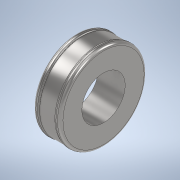
# Autodesk Inventor part: f8-16 thrust bearing
Saved by Autodesk Inventor 2020.4 (Build 244396000, 396)
## iProperties
Created: 2021-04-01
Part Number: f8-16 thrust bearing
Material: Stainless Steel
Document SubType Name: Modeling
Designer: AOB
Mass: 5.86086 g
Surface Area: 6.71687 cm^2
Volume: 0.732608 cm^3
Density: 8 g/cm^3
Appearance: Semi-Polished
Author: AOB
Autodesk Inventor part; units mm, degrees
ref_plane "YZ Plane" through (0, 0, 0) normal (1, 0, 0) x (0, 1, 0)
ref_plane "XZ Plane" through (0, 0, 0) normal (0, 1, 0) x (-1, 0, 0)
ref_plane "XY Plane" through (0, 0, 0) normal (0, 0, 1) x (1, 0, 0)
sketch "Sketch1" plane through (0, 0, 0) normal (0, 0, 1) x (1, 0, 0)
  line L0 (5, -0.5) -> (5, -4)
  line L1 (5, -4) -> (0, -4)
  line L2 (0, -4) -> (0, -0.5)
  arc A0 (0.5, 0) -> (0, -0.5) centre (0.5, -0.5) ccw
  arc A1 (5, -0.5) -> (4.5, 0) centre (4.5, -0.5) ccw
  line L3 (0.5, 0) -> (0.8, 0)
  line L4 (4.2, 0) -> (4.5, 0)
  arc A2 (1, -0.2) -> (0.8, 0) centre (0.8, -0.2) ccw
  arc A3 (4.2, 0) -> (4, -0.2) centre (4.2, -0.2) ccw
  line L5 (5, -4) -> (5, -8) construction
  line L6 (5, -8) -> (-0.4766, -8)
  line L7 (1.1, -0.1) -> (3.9, -0.1)
  line L8 (4, -0.2) -> (4, -0.2)
  arc A4 (4, -0.2) -> (3.9, -0.1) centre (3.9, -0.2) ccw
  line L9 (1, -0.2) -> (1, -0.2)
  arc A5 (1.1, -0.1) -> (1, -0.2) centre (1.1, -0.2) ccw
  point P0 (0, 0)
  point P1 (5, 0)
  point P2 (1.0268, -0.1)
  point P3 (3.9732, -0.1)
  point P4 (0.8978, 0)
  dimension "d0" = 5
  dimension "d1" = 4
  dimension "d2" = 0.5
  dimension "d4" = 0.2
  dimension "d5" = 4
  dimension "d9" = 0.1
  dimension "d10" = 0.1
  constraints: 20 end point, 13 point on circle, 10 tangent, 6 centre point, 6 point on line, 3 vertical, 2 equal radius, 2 perpendicular, 1 horizontal
  measures "d0" distance of point (0, 0) point (5, 0)
  measures "d1" distance of point (5, 0) L0.end
  measures "d2" radius of A0
  measures "d4" radius of A2
  measures "d5" distance of L0.end L5.end
  measures "d9" radius of A4
  measures "d10" radius of A5
revolve "Revolution1" add sketch "Sketch1" angle 360 about axis through (5, -8, 0) along (-1, 0, 0)
body "Solid1"
